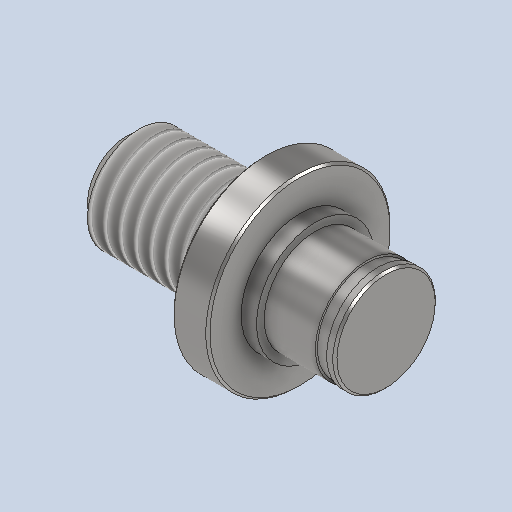
# Autodesk Inventor part: ParallelMecha_Gabel_Connection_JointShaft_Rillenkugellager
Saved by Autodesk Inventor 2024 (Build 280153000, 153)
## iProperties
Created: 2022-07-21
Part Number: ParallelMecha_Gabel_Connection_JointShaft_Rillenkugellager
Material: Edelstahl
Document SubType Name: Modeling
Designer: alexw
Density: 8 g/cm^3
Appearance: Halbpoliert
Mass: 20.9322 g
Surface Area: 13.7074 cm^2
Volume: 2.61652 cm^3
Flansch_Thickness: 3,500 mm
Gabel_FixationShaft_Contact_Thickness: 3,500 mm
Author: alexw
Autodesk Inventor part; units mm, degrees
ref_plane "YZ Plane" through (0, 0, 0) normal (1, 0, 0) x (0, 1, 0)
ref_plane "XZ Plane" through (0, 0, 0) normal (0, 1, 0) x (-1, 0, 0)
ref_plane "XY Plane" through (0, 0, 0) normal (0, 0, 1) x (1, 0, 0)
sketch "Skizze1" plane through (0, 0, 0) normal (0, 0, 1) x (1, 0, 0)
  line L0 (0, 0) -> (0, 9)
  line L1 (3.5, 9) -> (3.5, 5)
  line L2 (3.5, 5) -> (10, 5)
  line L3 (10, 5) -> (10, 4.8)
  line L4 (10, 4.8) -> (11.1, 4.8)
  line L5 (11.1, 4.8) -> (11.1, 5)
  line L6 (11.1, 5) -> (11.7, 5)
  line L7 (11.9, 4.8) -> (11.9, 0)
  line L8 (11.9, 0) -> (0, 0)
  line L9 (11.7, 5) -> (11.9, 4.8)
  line L10 (0, 5) -> (-13.5, 5)
  line L11 (-13.5, 5) -> (-13.5, 0)
  line L12 (-13.5, 0) -> (0, 0)
  line L13 (3.5, 9) -> (0, 9)
  line L14 (5, 5) -> (5, 0) construction
  line L15 (3.5, 5.75) -> (5, 5.75)
  line L16 (5, 5.75) -> (5, 5)
  point P0 (11.9, 5)
  dimension "d0" = 9.6
  dimension "d1" = 10
  dimension "d2" = 1.1
  dimension "d3" = 0.2
  dimension "d4" = 0.2
  dimension "d5" = 0.6
  dimension "Gabel_FixationShaft_Contact_Thickness" = 3.5
  dimension "d29" = 10
  dimension "d30" = 13.5
  dimension "d37" = 18
  dimension "d39" = 5
  dimension "d40" = 1.5
  dimension "d41" = 11.5
  constraints: 34 end point, 10 perpendicular, 9 point on line, 2 collinear, 1 horizontal, 1 vertical
  measures "d0" diameter of L4 L8
  measures "d1" diameter of L2 L8
  measures "d2" distance between parallel lines of L5 L3
  measures "d3" distance of L6.end point (11.9, 5)
  measures "d4" distance of L7.start point (11.9, 5)
  measures "d5" distance from line of L6.end L5
  measures "Gabel_FixationShaft_Contact_Thickness" distance between parallel lines of L0 L1
  measures "d29" diameter of L10 L12
  measures "d30" distance between parallel lines of L0 L11
  measures "d37" diameter of L13 L8
  measures "d39" distance between parallel lines of L3 L14
  measures "d40" distance between parallel lines of L14 L1
  measures "d41" diameter of L15 L8
revolve "Umdrehung1" add sketch "Skizze1" angle 360 about axis through (11.9, 0, 0) along (-1, 0, 0)
chamfer "Fase1" distance 0.2 angle 45 2 edges at (3.5, -9, 0) (0, -9, 0)
chamfer "Fase2" distance 1.25 angle 45 1 edges at (-13.5, -5, 0)
thread "Gewinde1" size "M10x1.5" class "6g" standard "ANSI Metric M Profile" full length
equation "\"d3\" = d4"
